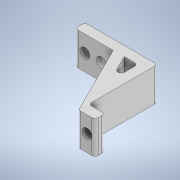
# Autodesk Inventor part: RightAngle_PulleySupport
Saved by Autodesk Inventor 2021 (Build 250183000, 183)
## iProperties
Created: 2021-11-23
Part Number: RightAngle_PulleySupport
Material: Generic
Document SubType Name: Modeling
Designer: Jorian Brusind
Density: 1 g/cm^3
Appearance: Default
Author: Jorian Brusind
Autodesk Inventor part; units mm, degrees
ref_plane "YZ Plane" through (0, 0, 0) normal (1, 0, 0) x (0, 1, 0)
ref_plane "XZ Plane" through (0, 0, 0) normal (0, 1, 0) x (-1, 0, 0)
ref_plane "XY Plane" through (0, 0, 0) normal (0, 0, 1) x (1, 0, 0)
sketch "Sketch1" plane through (0, 0, 0) normal (0, 1, 0) x (-1, 0, 0)
  line L0 (0, 0) -> (0, -48)
  line L1 (0, -48) -> (24, -48)
  line L2 (24, -48) -> (0, 0)
  line L3 (6, -25.4164) -> (6, -42)
  line L4 (6, -42) -> (14.2918, -42)
  line L5 (14.2918, -42) -> (6, -25.4164)
  line L6 (0, 0) -> (-10, 0)
  line L7 (-10, 0) -> (-10, -6)
  line L8 (-10, -6) -> (0, -6)
  line L9 (0, -6) -> (0, 0)
  dimension "d0" = 48
  dimension "d1" = 24
  dimension "d4" = 6
  dimension "d5" = 10
  dimension "d6" = 6
  constraints: 20 end point, 3 perpendicular, 2 parallel, 1 horizontal, 1 vertical, 2 other
  measures "d0" distance of L0.start L0.end
  measures "d1" distance of L0.end L1.end
  measures "d4" distance between parallel lines of L2 L5
  measures "d5" distance of L0.start L6.end
  measures "d6" distance of L7.end L6.end
extrude "Extrusion1" add sketch "Sketch1" along normal blind 20
sketch "Sketch2" plane through (0, 0, 0) normal (0, 0, 1) x (1, 0, 0)
  circle A0 centre (5, 10) radius 3
  line L0 (0, 0) -> (10, 0) projected
  line L1 (0, 0) -> (0, 20) projected
  dimension "d9" = 6
  dimension "d10" = 10
  dimension "d11" = 5
  constraints: 1 centre point
  measures "d9" diameter of A0
  measures "d10" distance from line of L0 A0.centre
  measures "d11" distance from line of L1 A0.centre
extrude "Extrusion2" cut sketch "Sketch2" against normal through all
sketch "Sketch3" plane through (0, 0, 0) normal (0, -1, 0) x (1, 0, 0)
  line L0 (-14.2918, -42) -> (-6, -42) projected
  line L1 (-14.2918, -42) -> (-44.2918, -42)
  line L2 (-44.2918, -42) -> (-19.2918, -42)
  line L3 (-19.2918, -42) -> (-19.2918, -48)
  line L4 (-19.2918, -48) -> (-44.2918, -48)
  line L5 (-44.2918, -48) -> (-44.2918, -42)
  point P0 (0, 0)
  dimension "d14" = 30
  dimension "d15" = 25
  dimension "d16" = 6
  constraints: 10 end point, 2 horizontal, 2 parallel, 1 perpendicular
  measures "d14" distance of L0.start L1.end
  measures "d15" distance of L3.end L4.end
  measures "d16" distance of L2.end L3.end
extrude "Extrusion3" add sketch "Sketch3" against normal blind 20
sketch "Sketch4" plane through (0, 0, -48) normal (0, 0, -1) x (-1, 0, 0)
  circle A0 centre (38.2918, 10) radius 3
  circle A1 centre (28.2918, 10) radius 3
  line L0 (44.2918, 0) -> (44.2918, 20) projected
  line L1 (0, 0) -> (44.2918, 0) projected
  dimension "d19" = 6
  dimension "d20" = 6
  dimension "d21" = 6
  dimension "d22" = 10
  dimension "d23" = 10
  dimension "d24" = 10
  constraints: 2 centre point
  measures "d19" diameter of A0
  measures "d20" diameter of A1
  measures "d21" distance from line of L0 A0.centre
  measures "d22" distance of A0.centre A1.centre
  measures "d23" distance from line of L1 A1.centre
  measures "d24" distance from line of L1 A0.centre
extrude "Extrusion4" cut sketch "Sketch4" against normal through all
fillet "Fillet1" radius 2 2 edges at (-6, 10, -42) (-6, 10, -25.4164)
fillet "Fillet2" radius 2 3 edges at (0, 10, -48) (-44.2918, 10, -48) (-44.2918, 10, -42)
fillet "Fillet3" radius 2 1 edges at (0, 10, -6)
fillet "Fillet4" radius 2 3 edges at (10, 10, 0) (10, 10, -6) (0, 10, 0)
body "Solid1"
